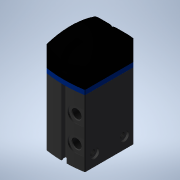
# Autodesk Inventor part: 1310164 DHRS-32-A---(Geh)
Saved by Autodesk Inventor 2025.1 (Build 291241000, 241)
## iProperties
Category: PARTsolutions
Company: FESTO
Created: 2025-06-16
Part Number: 1310164 DHRS-32-A---(Geh)
Material: Generic
Catalog Web Link: www.cadenas.de
Description: DHRS---(Geh)-Housing
Vendor: FESTO
Document SubType Name: Modeling
Designer: psAdmin
Manufacturer: FESTO
Mass: 163.482 g
Surface Area: 252.233 cm^2
Volume: 163.482 cm^3
Density: 1 g/cm^3
Appearance: PSOLRGB-175-175-175
PSOL_IDENT_0: {$CADENAS_DATA/23d-libs/festo/parts/d/dhrs/parts/dhrs_geh.prj},196 {VTYP=3D},{NB=1310164 DHRS-32-A--
PSOL_IDENT_1: -(Geh)},{LINA=1310164 DHRS-32-A---(Geh)},{NN=DHRS---(Geh)},{DATE=04.06.2025 19:34:44},{GEOMDATE=22.0
PSOL_IDENT_2: 8.2023 11:13:58},{VERSION=},{LINEID=60},{WBVAR=},{WBNUMERIC=}  {NB=1310164 DHRS-32-A---(Geh)},{LINA=
PSOL_IDENT_3: 1310164 DHRS-32-A---(Geh)},{KT=DUMMY},{TNR=1310164},{TYP=DHRS-32-A},{GR=32}
NB: 1310164 DHRS-32-A---(Geh)
NN: DHRS---(Geh)
NT: Housing
NBSYN: $TNR. $TYP.---(Geh)
LINA: 1310164 DHRS-32-A---(Geh)
CATALOG: Festo
TNR: 1310164
TYP: DHRS-32-A
GR: 32
SUPPLIER: FESTO
ARTICLENO: 1310164 DHRS-32-A---(Geh)
BOMINFO: 1310164 DHRS-32-A---(Geh)
CREATOR: CADENAS GmbH
Title: 1310164 DHRS-32-A---(Geh)
Author: Cadenas PARTsolutions
Comments: Housing
Autodesk Inventor part; units mm, degrees
sketch "Sketch_1" plane through (0, 0, 0) normal (0, 1, 0) x (-1, 0, 0)
  line L0 (19, -23.0657) -> (19, 23.0657)
  arc A0 (19, 23.0657) -> (18.1678, 24.043) centre (18.01, 23.0657) ccw
  arc A1 (18.1678, 24.043) -> (2.6, 25.4703) centre (0, -88.5) ccw
  line L1 (2.6, 25.4703) -> (2.6, 23.9)
  line L2 (2.6, 23.9) -> (3.25, 23.9)
  line L3 (3.25, 23.9) -> (3.25, 20.7)
  line L4 (3.25, 20.7) -> (-3.25, 20.7)
  line L5 (-3.25, 20.7) -> (-3.25, 23.9)
  line L6 (-3.25, 23.9) -> (-2.6, 23.9)
  line L7 (-2.6, 23.9) -> (-2.6, 25.4703)
  arc A2 (-2.6, 25.4703) -> (-18.1678, 24.043) centre (0, -88.5) ccw
  arc A3 (-18.1678, 24.043) -> (-19, 23.0657) centre (-18.01, 23.0657) ccw
  line L8 (-19, 23.0657) -> (-19, -23.0657)
  arc A4 (-19, -23.0657) -> (-18.1678, -24.043) centre (-18.01, -23.0657) ccw
  arc A5 (-18.1678, -24.043) -> (-2.6, -25.4703) centre (0, 88.5) ccw
  line L9 (-2.6, -25.4703) -> (-2.6, -23.9)
  line L10 (-2.6, -23.9) -> (-3.25, -23.9)
  line L11 (-3.25, -23.9) -> (-3.25, -20.7)
  line L12 (-3.25, -20.7) -> (3.25, -20.7)
  line L13 (3.25, -20.7) -> (3.25, -23.9)
  line L14 (3.25, -23.9) -> (2.6, -23.9)
  line L15 (2.6, -23.9) -> (2.6, -25.4703)
  arc A6 (2.6, -25.4703) -> (18.1678, -24.043) centre (0, 88.5) ccw
  arc A7 (18.1678, -24.043) -> (19, -23.0657) centre (18.01, -23.0657) ccw
  constraints: 32 end point, 16 point on circle, 8 centre point
extrude "Extrusion1" add sketch "Sketch_1" along normal blind 65
sketch "Sketch_2" plane through (0, 69.5, 0) normal (0, 1, 0) x (1, 0, 0)
  line L0 (-18.905, 22.961) -> (-18.905, -22.961)
  arc A0 (-18.905, -22.961) -> (-18.0636, -23.9484) centre (-17.905, -22.961) ccw
  arc A1 (-18.0636, -23.9484) -> (18.0636, -23.9484) centre (0, 88.5) ccw
  arc A2 (18.0636, -23.9484) -> (18.905, -22.961) centre (17.905, -22.961) ccw
  line L1 (18.905, -22.961) -> (18.905, 22.961)
  arc A3 (18.905, 22.961) -> (18.0636, 23.9484) centre (17.905, 22.961) ccw
  arc A4 (18.0636, 23.9484) -> (-18.0636, 23.9484) centre (0, -88.5) ccw
  arc A5 (-18.0636, 23.9484) -> (-18.905, 22.961) centre (-17.905, 22.961) ccw
  constraints: 12 point on circle, 6 centre point, 4 end point
extrude "Extrusion2" add sketch "Sketch_2" against normal blind 4.5
sketch "Sketch_3" plane through (0, 69.5, 0) normal (0, 1, 0) x (1, 0, 0)
  line L0 (-18.925, 22.9882) -> (-18.925, -22.9882)
  arc A0 (-18.925, -22.9882) -> (-18.0837, -23.9755) centre (-17.925, -22.9882) ccw
  arc A1 (-18.0837, -23.9755) -> (18.0837, -23.9755) centre (0, 88.5) ccw
  arc A2 (18.0837, -23.9755) -> (18.925, -22.9882) centre (17.925, -22.9882) ccw
  line L1 (18.925, -22.9882) -> (18.925, 22.9882)
  arc A3 (18.925, 22.9882) -> (18.0837, 23.9755) centre (17.925, 22.9882) ccw
  arc A4 (18.0837, 23.9755) -> (-18.0837, 23.9755) centre (0, -88.5) ccw
  arc A5 (-18.0837, 23.9755) -> (-18.925, 22.9882) centre (-17.925, 22.9882) ccw
  constraints: 12 point on circle, 6 centre point, 4 end point
extrude "Extrusion3" add sketch "Sketch_3" along normal blind 30
sketch "Sketch_4" plane through (0, 0, 0) normal (0, 0, 1) x (1, 0, 0)
  line L0 (20, 19.7) -> (-20, 19.7)
  arc A0 (25, 90.425) -> (-25, 90.425) centre (0, 39.2) ccw
  line L1 (25, 90.425) -> (25, 115)
  line L2 (25, 115) -> (-25, 115)
  line L3 (-25, 115) -> (-25, 90.425)
  constraints: 8 end point, 2 point on circle, 1 centre point
revolve "Revolution1" cut sketch "Sketch_4" angle 60 mid plane about axis through (20, 19.7, 0) along (-1, 0, 0)
sketch "Sketch_5" plane through (0, 0, 0) normal (1, 0, 0) x (0, 1, 0)
  line L0 (83.6055, 30.41) -> (83.6055, 25.41)
  arc A0 (94.3361, 16.8296) -> (83.6055, 25.41) centre (83.6055, 14.41) ccw
  arc A1 (94.3361, -16.8296) -> (94.3361, 16.8296) centre (19.7, 0) ccw
  arc A2 (83.6055, -25.41) -> (94.3361, -16.8296) centre (83.6055, -14.41) ccw
  line L1 (83.6055, -25.41) -> (83.6055, -30.41)
  line L2 (83.6055, -30.41) -> (110, -30.41)
  line L3 (110, -30.41) -> (110, 30.41)
  line L4 (110, 30.41) -> (83.6055, 30.41)
  constraints: 10 end point, 6 point on circle, 3 centre point
extrude "Extrusion4" cut sketch "Sketch_5" along normal mid plane 50
sketch "Sketch_7" plane through (0, 74.7, 0) normal (0, 1, 0) x (1, 0, 0)
  line L0 (-3, -9.7035) -> (-3, -30)
  line L1 (-3, -30) -> (3, -30)
  line L2 (3, -30) -> (3, -9.7035)
  arc A0 (-3, -9.7035) -> (3, -9.7035) centre (0, 13.1) ccw
  constraints: 6 end point, 2 point on circle, 1 centre point
extrude "Extrusion5" cut sketch "Sketch_7" along normal blind 25
sketch "Sketch_19" plane through (0, 74.7, 0) normal (0, 1, 0) x (1, 0, 0)
  arc A0 (3, 9.7035) -> (-3, 9.7035) centre (0, -13.1) ccw
  line L0 (3, 9.7035) -> (3, 30)
  line L1 (3, 30) -> (-3, 30)
  line L2 (-3, 30) -> (-3, 9.7035)
  constraints: 6 end point, 2 point on circle, 1 centre point
extrude "Extrusion6" cut sketch "Sketch_19" along normal blind 25
sketch "Sketch_6" plane through (0, 0, 0) normal (1, 0, 0) x (0, 1, 0)
  circle A0 centre (82.5, 12.9) radius 12.6
  constraints: 1 centre point
extrude "Extrusion7" cut sketch "Sketch_6" along normal mid plane 6
sketch "Sketch_17" plane through (0, 0, 0) normal (1, 0, 0) x (0, 1, 0)
  circle A0 centre (82.5, -12.9) radius 12.6
  constraints: 1 centre point
extrude "Extrusion8" cut sketch "Sketch_17" along normal mid plane 6
sketch "Sketch_10" plane through (0, 0, 24.044) normal (0, 0, 1) x (1, 0, 0)
  arc A0 (11, 52.5) -> (11, 37.5) centre (11, 45) ccw
  line L0 (11, 37.5) -> (21, 37.5)
  line L1 (21, 37.5) -> (21, 27.5)
  line L2 (21, 27.5) -> (11, 27.5)
  arc A1 (11, 27.5) -> (11, 12.5) centre (11, 20) ccw
  line L3 (11, 12.5) -> (26, 12.5)
  line L4 (26, 12.5) -> (26, 52.5)
  line L5 (26, 52.5) -> (11, 52.5)
  constraints: 12 end point, 4 point on circle, 2 centre point
extrude "Extrusion9" cut sketch "Sketch_10" along normal blind 3
sketch "Sketch11" plane through (0, 0, 24.044) normal (0, 0, 1) x (1, 0, 0)
  point P0 (11, 20)
hole "Hole1" at (11, 20, 24.044) direction (0, 0, -1) diameter 8.566 depth 7.5 countersink diameter 9.728 countersink angle 90 thread size "G9.728x0.907" designation "G 1/8" standard "ISO Pipe Threads"
sketch "Sketch12" plane through (0, 0, 24.044) normal (0, 0, 1) x (1, 0, 0)
  point P0 (11, 45)
hole "Hole2" at (11, 45, 24.044) direction (0, 0, -1) diameter 8.566 depth 7.5 countersink diameter 9.728 countersink angle 90 thread size "G9.728x0.907" designation "G 1/8" standard "ISO Pipe Threads"
sketch "Sketch13" plane through (-19, 0, -23.0657) normal (-1, 0, 0) x (0, 0, 1)
  point P0 (37.5657, 11)
hole "Hole3" at (-19, 11, 14.5) direction (1, 0, 0) diameter 4.917 depth 19 counterbore diameter 9 counterbore depth 2.1 thread size "M6x1" class "6H" standard "ISO Metric profile"
sketch "Sketch14" plane through (19, 0, 23.0657) normal (1, 0, 0) x (0, 0, -1)
  point P0 (8.5657, 11)
hole "Hole4" at (19, 11, 14.5) direction (-1, 0, 0) diameter 4.917 depth 19 counterbore diameter 9 counterbore depth 2.1 thread size "M6x1" class "6H" standard "ISO Metric profile"
sketch "Sketch15" plane through (-19, 0, -23.0657) normal (-1, 0, 0) x (0, 0, 1)
  point P0 (8.5657, 11)
hole "Hole5" at (-19, 11, -14.5) direction (1, 0, 0) diameter 4.917 depth 19 counterbore diameter 9 counterbore depth 2.1 thread size "M6x1" class "6H" standard "ISO Metric profile"
sketch "Sketch16" plane through (19, 0, 23.0657) normal (1, 0, 0) x (0, 0, -1)
  point P0 (37.5657, 11)
hole "Hole6" at (19, 11, -14.5) direction (-1, 0, 0) diameter 4.917 depth 19 counterbore diameter 9 counterbore depth 2.1 thread size "M6x1" class "6H" standard "ISO Metric profile"
sketch "Sketch17" plane through (0, 0, 0) normal (0, -1, 0) x (1, 0, 0)
  point P0 (0, 14.5)
hole "Hole7" at (0, 0, 14.5) direction (0, 1, 0) diameter 4.917 depth 11 counterbore diameter 9 counterbore depth 2.1 thread size "M6x1" class "6H" standard "ISO Metric profile"
sketch "Sketch18" plane through (0, 0, 0) normal (0, -1, 0) x (1, 0, 0)
  point P0 (0, -14.5)
hole "Hole8" at (0, 0, -14.5) direction (0, 1, 0) diameter 4.917 depth 11 counterbore diameter 9 counterbore depth 2.1 thread size "M6x1" class "6H" standard "ISO Metric profile"
sketch "Sketch_22" plane through (0, 0, 0) normal (1, 0, 0) x (0, 1, 0)
  arc A0 (71.2251, 20.505) -> (76.3257, 0.7823) centre (82.5, 12.9) ccw
  line L0 (76.3257, 0.7823) -> (82.5, 12.9)
  line L1 (82.5, 12.9) -> (71.2251, 20.505)
  constraints: 4 end point, 2 point on circle, 1 centre point
extrude "Extrusion10" cut sketch "Sketch_22" along normal mid plane 2
sketch "Sketch_23" plane through (0, 0, 0) normal (1, 0, 0) x (0, 1, 0)
  arc A0 (76.3257, -0.7823) -> (71.2251, -20.505) centre (82.5, -12.9) ccw
  line L0 (71.2251, -20.505) -> (82.5, -12.9)
  line L1 (82.5, -12.9) -> (76.3257, -0.7823)
  constraints: 4 end point, 2 point on circle, 1 centre point
extrude "Extrusion11" cut sketch "Sketch_23" along normal mid plane 2
ref_plane "GEHAEUSE_XY" through (0, 0, 0) normal (0, 1, 0) x (1, 0, 0)
ref_plane "GEHAEUSE_YZ" through (0, 0, 0) normal (1, 0, 0) x (0, 0, -1)
ref_plane "GEHAEUSE_ZX" through (0, 0, 0) normal (0, 0, -1) x (0, 1, 0)
ref_plane "TO_JAW_L_XY" through (0, 82.5, 12.9) normal (1, 0, 0) x (0, 0, -1)
ref_plane "TO_JAW_L_YZ" through (0, 82.5, 12.9) normal (0, 0, -1) x (0, 1, 0)
ref_plane "TO_JAW_L_ZX" through (0, 82.5, 12.9) normal (0, 1, 0) x (1, 0, 0)
ref_plane "TO_JAW_R_XY" through (0, 82.5, -12.9) normal (1, 0, 0) x (0, 0, -1)
ref_plane "TO_JAW_R_YZ" through (0, 82.5, -12.9) normal (0, 0, -1) x (0, 1, 0)
ref_plane "TO_JAW_R_ZX" through (0, 82.5, -12.9) normal (0, 1, 0) x (1, 0, 0)
ref_plane "TO_ZBH_1_XY" through (0, 2.1, -14.5) normal (0, 1, 0) x (1, 0, 0)
ref_plane "TO_ZBH_1_YZ" through (0, 2.1, -14.5) normal (1, 0, 0) x (0, 0, -1)
ref_plane "TO_ZBH_1_ZX" through (0, 2.1, -14.5) normal (0, 0, -1) x (0, 1, 0)
ref_plane "TO_ZBH_2_XY" through (0, 2.1, 14.5) normal (0, 1, 0) x (1, 0, 0)
ref_plane "TO_ZBH_2_YZ" through (0, 2.1, 14.5) normal (1, 0, 0) x (0, 0, -1)
ref_plane "TO_ZBH_2_ZX" through (0, 2.1, 14.5) normal (0, 0, -1) x (0, 1, 0)
body "Solid1"
